Trimix_Enclosure_A1 (Autodesk Fusion 360 design; units mm, degrees)
Autodesk Fusion 360 part; units mm, degrees
(part 1 of 3)
ref_plane "WorkPlane1" through (0, 0, 0) normal (0, 0, 1) x (1, 0, 0) in component "01 Main housing"
sketch "Main housing sketch" plane through (0, 0, 0) normal (0, 0, 1) x (1, 0, 0) in component "01 Main housing"
  line L0 (-47.5, 0) -> (47.5, 0)
  line L1 (47.5, 0) -> (47.5, 180)
  line L2 (47.5, 180) -> (-47.5, 180)
  line L3 (-47.5, 180) -> (-47.5, 0)
  dimension "d42" = 47.5
  dimension "d43" = 95
  dimension "d44" = 180
  constraint horizontal origin L0.start
  constraint horizontal L0
  constraint vertical L1
  constraint horizontal L2
  constraint vertical L3
  measures "d42" horizontal distance of origin L0.start
  measures "d43" horizontal distance of L0.start L0.end
  measures "d44" vertical distance of L0.end L1.end
extrude "Main housing" add sketch "Main housing sketch" along normal blind 57 makes body 1 in component "01 Main housing"
fillet "Outside corner rounds" radius 8 4 edges at (-47.5, 180, 28.5) (47.5, 180, 28.5) (47.5, 0, 28.5) (-47.5, 0, 28.5) on bodies 1 in component "01 Main housing"
ref_plane "WorkPlane2" through (0, 0, 3) normal (0, 0, 1) x (1, 0, 0) in component "01 Main housing"
sketch "Rear-open cavity sketch" plane through (0, 0, 3) normal (0, 0, 1) x (1, 0, 0) in component "01 Main housing"
  line L0 (-44.5, 3) -> (44.5, 3)
  line L1 (44.5, 3) -> (44.5, 177)
  line L2 (44.5, 177) -> (-44.5, 177)
  line L3 (-44.5, 177) -> (-44.5, 3)
  dimension "d51" = 44.5
  dimension "d52" = 3
  dimension "d53" = 89
  dimension "d54" = 174
  constraint horizontal L0
  constraint vertical L1
  constraint horizontal L2
  constraint vertical L3
  measures "d51" horizontal distance of origin L0.start
  measures "d52" vertical distance of origin L0.start
  measures "d53" horizontal distance of L0.start L0.end
  measures "d54" vertical distance of L0.end L1.end
extrude "Rear-open cavity" cut sketch "Rear-open cavity sketch" along normal blind 60 bodies 1 in component "01 Main housing"
fillet "Inside corner rounds" radius 5 4 edges at (44.5, 3, 30) (-44.5, 3, 30) (-44.5, 177, 30) (44.5, 177, 30) on bodies 1 in component "01 Main housing"
ref_plane "WorkPlane3" through (0, 0, -1) normal (0, 0, 1) x (1, 0, 0) in component "01 Main housing"
sketch "Screen aperture sketch" plane through (0, 0, -1) normal (0, 0, 1) x (1, 0, 0) in component "01 Main housing"
  line L0 (-28.58, 21.205) -> (28.58, 21.205)
  line L1 (28.58, 21.205) -> (28.58, 115.805)
  line L2 (28.58, 115.805) -> (-28.58, 115.805)
  line L3 (-28.58, 115.805) -> (-28.58, 21.205)
  dimension "d61" = 28.58
  dimension "d62" = 21.205
  dimension "d63" = 57.16
  dimension "d64" = 94.6
  constraint horizontal L0
  constraint vertical L1
  constraint horizontal L2
  constraint vertical L3
  measures "d61" horizontal distance of origin L0.start
  measures "d62" vertical distance of origin L0.start
  measures "d63" horizontal distance of L0.start L0.end
  measures "d64" vertical distance of L0.end L1.end
extrude "Screen aperture" cut sketch "Screen aperture sketch" along normal blind 5 bodies 1 in component "01 Main housing"
ref_plane "WorkPlane4" through (0, 0, 3) normal (0, 0, 1) x (1, 0, 0) in component "01 Main housing"
sketch "Boss -1_0 sketch" plane through (0, 0, 3) normal (0, 0, 1) x (1, 0, 0) in component "01 Main housing"
  circle A0 centre (-40, 8) radius 4.5
  dimension "d69" = 40
  dimension "d70" = 8
  dimension "d71" = 4.5
  measures "d69" horizontal distance of origin A0.centre
  measures "d70" vertical distance of origin A0.centre
  measures "d71" radius of A0
extrude "Boss -1_0" add sketch "Boss -1_0 sketch" along normal blind 54 bodies 1 in component "01 Main housing"
ref_plane "WorkPlane5" through (0, 0, 3) normal (0, 0, 1) x (1, 0, 0) in component "01 Main housing"
sketch "Boss web -1_0 sketch" plane through (0, 0, 3) normal (0, 0, 1) x (1, 0, 0) in component "01 Main housing"
  line L0 (-44.5, 3.5) -> (-40, 3.5)
  line L1 (-40, 3.5) -> (-40, 12.5)
  line L2 (-40, 12.5) -> (-44.5, 12.5)
  line L3 (-44.5, 12.5) -> (-44.5, 3.5)
  dimension "d76" = 44.5
  dimension "d77" = 3.5
  dimension "d78" = 4.5
  dimension "d79" = 9
  constraint horizontal L0
  constraint vertical L1
  constraint horizontal L2
  constraint vertical L3
  measures "d76" horizontal distance of origin L0.start
  measures "d77" vertical distance of origin L0.start
  measures "d78" horizontal distance of L0.start L0.end
  measures "d79" vertical distance of L0.end L1.end
extrude "Boss web -1_0" add sketch "Boss web -1_0 sketch" along normal blind 54 bodies 1 in component "01 Main housing"
ref_plane "WorkPlane6" through (0, 0, 52) normal (0, 0, 1) x (1, 0, 0) in component "01 Main housing"
sketch "Insert pilot -1_0 sketch" plane through (0, 0, 52) normal (0, 0, 1) x (1, 0, 0) in component "01 Main housing"
  circle A0 centre (-40, 8) radius 2.1
  dimension "d84" = 40
  dimension "d85" = 8
  dimension "d86" = 2.1
  measures "d84" horizontal distance of origin A0.centre
  measures "d85" vertical distance of origin A0.centre
  measures "d86" radius of A0
extrude "Insert pilot -1_0" cut sketch "Insert pilot -1_0 sketch" along normal blind 5.1 bodies 1 in component "01 Main housing"
ref_plane "WorkPlane7" through (0, 0, 3) normal (0, 0, 1) x (1, 0, 0) in component "01 Main housing"
sketch "Boss -1_1 sketch" plane through (0, 0, 3) normal (0, 0, 1) x (1, 0, 0) in component "01 Main housing"
  circle A0 centre (-40, 90) radius 4.5
  dimension "d91" = 40
  dimension "d92" = 90
  dimension "d93" = 4.5
  measures "d91" horizontal distance of origin A0.centre
  measures "d92" vertical distance of origin A0.centre
  measures "d93" radius of A0
extrude "Boss -1_1" add sketch "Boss -1_1 sketch" along normal blind 54 bodies 1 in component "01 Main housing"
ref_plane "WorkPlane8" through (0, 0, 3) normal (0, 0, 1) x (1, 0, 0) in component "01 Main housing"
sketch "Boss web -1_1 sketch" plane through (0, 0, 3) normal (0, 0, 1) x (1, 0, 0) in component "01 Main housing"
  line L0 (-44.5, 85.5) -> (-40, 85.5)
  line L1 (-40, 85.5) -> (-40, 94.5)
  line L2 (-40, 94.5) -> (-44.5, 94.5)
  line L3 (-44.5, 94.5) -> (-44.5, 85.5)
  dimension "d98" = 44.5
  dimension "d99" = 85.5
  dimension "d100" = 4.5
  dimension "d101" = 9
  constraint horizontal L0
  constraint vertical L1
  constraint horizontal L2
  constraint vertical L3
  measures "d98" horizontal distance of origin L0.start
  measures "d99" vertical distance of origin L0.start
  measures "d100" horizontal distance of L0.start L0.end
  measures "d101" vertical distance of L0.end L1.end
extrude "Boss web -1_1" add sketch "Boss web -1_1 sketch" along normal blind 54 bodies 1 in component "01 Main housing"
ref_plane "WorkPlane9" through (0, 0, 52) normal (0, 0, 1) x (1, 0, 0) in component "01 Main housing"
sketch "Insert pilot -1_1 sketch" plane through (0, 0, 52) normal (0, 0, 1) x (1, 0, 0) in component "01 Main housing"
  circle A0 centre (-40, 90) radius 2.1
  dimension "d106" = 40
  dimension "d107" = 90
  dimension "d108" = 2.1
  measures "d106" horizontal distance of origin A0.centre
  measures "d107" vertical distance of origin A0.centre
  measures "d108" radius of A0
extrude "Insert pilot -1_1" cut sketch "Insert pilot -1_1 sketch" along normal blind 5.1 bodies 1 in component "01 Main housing"
ref_plane "WorkPlane10" through (0, 0, 3) normal (0, 0, 1) x (1, 0, 0) in component "01 Main housing"
sketch "Boss -1_2 sketch" plane through (0, 0, 3) normal (0, 0, 1) x (1, 0, 0) in component "01 Main housing"
  circle A0 centre (-40, 172) radius 4.5
  dimension "d113" = 40
  dimension "d114" = 172
  dimension "d115" = 4.5
  measures "d113" horizontal distance of origin A0.centre
  measures "d114" vertical distance of origin A0.centre
  measures "d115" radius of A0
extrude "Boss -1_2" add sketch "Boss -1_2 sketch" along normal blind 54 bodies 1 in component "01 Main housing"
ref_plane "WorkPlane11" through (0, 0, 3) normal (0, 0, 1) x (1, 0, 0) in component "01 Main housing"
sketch "Boss web -1_2 sketch" plane through (0, 0, 3) normal (0, 0, 1) x (1, 0, 0) in component "01 Main housing"
  line L0 (-44.5, 167.5) -> (-40, 167.5)
  line L1 (-40, 167.5) -> (-40, 176.5)
  line L2 (-40, 176.5) -> (-44.5, 176.5)
  line L3 (-44.5, 176.5) -> (-44.5, 167.5)
  dimension "d120" = 44.5
  dimension "d121" = 167.5
  dimension "d122" = 4.5
  dimension "d123" = 9
  constraint horizontal L0
  constraint vertical L1
  constraint horizontal L2
  constraint vertical L3
  measures "d120" horizontal distance of origin L0.start
  measures "d121" vertical distance of origin L0.start
  measures "d122" horizontal distance of L0.start L0.end
  measures "d123" vertical distance of L0.end L1.end
extrude "Boss web -1_2" add sketch "Boss web -1_2 sketch" along normal blind 54 bodies 1 in component "01 Main housing"
ref_plane "WorkPlane12" through (0, 0, 52) normal (0, 0, 1) x (1, 0, 0) in component "01 Main housing"
sketch "Insert pilot -1_2 sketch" plane through (0, 0, 52) normal (0, 0, 1) x (1, 0, 0) in component "01 Main housing"
  circle A0 centre (-40, 172) radius 2.1
  dimension "d128" = 40
  dimension "d129" = 172
  dimension "d130" = 2.1
  measures "d128" horizontal distance of origin A0.centre
  measures "d129" vertical distance of origin A0.centre
  measures "d130" radius of A0
extrude "Insert pilot -1_2" cut sketch "Insert pilot -1_2 sketch" along normal blind 5.1 bodies 1 in component "01 Main housing"
ref_plane "WorkPlane13" through (0, 0, 3) normal (0, 0, 1) x (1, 0, 0) in component "01 Main housing"
sketch "Boss 1_0 sketch" plane through (0, 0, 3) normal (0, 0, 1) x (1, 0, 0) in component "01 Main housing"
  circle A0 centre (40, 8) radius 4.5
  dimension "d135" = 40
  dimension "d136" = 8
  dimension "d137" = 4.5
  measures "d135" horizontal distance of origin A0.centre
  measures "d136" vertical distance of origin A0.centre
  measures "d137" radius of A0
extrude "Boss 1_0" add sketch "Boss 1_0 sketch" along normal blind 54 bodies 1 in component "01 Main housing"
ref_plane "WorkPlane14" through (0, 0, 3) normal (0, 0, 1) x (1, 0, 0) in component "01 Main housing"
sketch "Boss web 1_0 sketch" plane through (0, 0, 3) normal (0, 0, 1) x (1, 0, 0) in component "01 Main housing"
  line L0 (40, 3.5) -> (44.5, 3.5)
  line L1 (44.5, 3.5) -> (44.5, 12.5)
  line L2 (44.5, 12.5) -> (40, 12.5)
  line L3 (40, 12.5) -> (40, 3.5)
  dimension "d142" = 40
  dimension "d143" = 3.5
  dimension "d144" = 4.5
  dimension "d145" = 9
  constraint horizontal L0
  constraint vertical L1
  constraint horizontal L2
  constraint vertical L3
  measures "d142" horizontal distance of origin L0.start
  measures "d143" vertical distance of origin L0.start
  measures "d144" horizontal distance of L0.start L0.end
  measures "d145" vertical distance of L0.end L1.end
extrude "Boss web 1_0" add sketch "Boss web 1_0 sketch" along normal blind 54 bodies 1 in component "01 Main housing"
ref_plane "WorkPlane15" through (0, 0, 52) normal (0, 0, 1) x (1, 0, 0) in component "01 Main housing"
sketch "Insert pilot 1_0 sketch" plane through (0, 0, 52) normal (0, 0, 1) x (1, 0, 0) in component "01 Main housing"
  circle A0 centre (40, 8) radius 2.1
  dimension "d150" = 40
  dimension "d151" = 8
  dimension "d152" = 2.1
  measures "d150" horizontal distance of origin A0.centre
  measures "d151" vertical distance of origin A0.centre
  measures "d152" radius of A0
extrude "Insert pilot 1_0" cut sketch "Insert pilot 1_0 sketch" along normal blind 5.1 bodies 1 in component "01 Main housing"
ref_plane "WorkPlane16" through (0, 0, 3) normal (0, 0, 1) x (1, 0, 0) in component "01 Main housing"
sketch "Boss 1_1 sketch" plane through (0, 0, 3) normal (0, 0, 1) x (1, 0, 0) in component "01 Main housing"
  circle A0 centre (40, 90) radius 4.5
  dimension "d157" = 40
  dimension "d158" = 90
  dimension "d159" = 4.5
  measures "d157" horizontal distance of origin A0.centre
  measures "d158" vertical distance of origin A0.centre
  measures "d159" radius of A0
extrude "Boss 1_1" add sketch "Boss 1_1 sketch" along normal blind 54 bodies 1 in component "01 Main housing"
ref_plane "WorkPlane17" through (0, 0, 3) normal (0, 0, 1) x (1, 0, 0) in component "01 Main housing"
sketch "Boss web 1_1 sketch" plane through (0, 0, 3) normal (0, 0, 1) x (1, 0, 0) in component "01 Main housing"
  line L0 (40, 85.5) -> (44.5, 85.5)
  line L1 (44.5, 85.5) -> (44.5, 94.5)
  line L2 (44.5, 94.5) -> (40, 94.5)
  line L3 (40, 94.5) -> (40, 85.5)
  dimension "d164" = 40
  dimension "d165" = 85.5
  dimension "d166" = 4.5
  dimension "d167" = 9
  constraint horizontal L0
  constraint vertical L1
  constraint horizontal L2
  constraint vertical L3
  measures "d164" horizontal distance of origin L0.start
  measures "d165" vertical distance of origin L0.start
  measures "d166" horizontal distance of L0.start L0.end
  measures "d167" vertical distance of L0.end L1.end
extrude "Boss web 1_1" add sketch "Boss web 1_1 sketch" along normal blind 54 bodies 1 in component "01 Main housing"
ref_plane "WorkPlane18" through (0, 0, 52) normal (0, 0, 1) x (1, 0, 0) in component "01 Main housing"
sketch "Insert pilot 1_1 sketch" plane through (0, 0, 52) normal (0, 0, 1) x (1, 0, 0) in component "01 Main housing"
  circle A0 centre (40, 90) radius 2.1
  dimension "d172" = 40
  dimension "d173" = 90
  dimension "d174" = 2.1
  measures "d172" horizontal distance of origin A0.centre
  measures "d173" vertical distance of origin A0.centre
  measures "d174" radius of A0
extrude "Insert pilot 1_1" cut sketch "Insert pilot 1_1 sketch" along normal blind 5.1 bodies 1 in component "01 Main housing"
ref_plane "WorkPlane19" through (0, 0, 3) normal (0, 0, 1) x (1, 0, 0) in component "01 Main housing"
sketch "Boss 1_2 sketch" plane through (0, 0, 3) normal (0, 0, 1) x (1, 0, 0) in component "01 Main housing"
  circle A0 centre (40, 172) radius 4.5
  dimension "d179" = 40
  dimension "d180" = 172
  dimension "d181" = 4.5
  measures "d179" horizontal distance of origin A0.centre
  measures "d180" vertical distance of origin A0.centre
  measures "d181" radius of A0
extrude "Boss 1_2" add sketch "Boss 1_2 sketch" along normal blind 54 bodies 1 in component "01 Main housing"
ref_plane "WorkPlane20" through (0, 0, 3) normal (0, 0, 1) x (1, 0, 0) in component "01 Main housing"
sketch "Boss web 1_2 sketch" plane through (0, 0, 3) normal (0, 0, 1) x (1, 0, 0) in component "01 Main housing"
  line L0 (40, 167.5) -> (44.5, 167.5)
  line L1 (44.5, 167.5) -> (44.5, 176.5)
  line L2 (44.5, 176.5) -> (40, 176.5)
  line L3 (40, 176.5) -> (40, 167.5)
  dimension "d186" = 40
  dimension "d187" = 167.5
  dimension "d188" = 4.5
  dimension "d189" = 9
  constraint horizontal L0
  constraint vertical L1
  constraint horizontal L2
  constraint vertical L3
  measures "d186" horizontal distance of origin L0.start
  measures "d187" vertical distance of origin L0.start
  measures "d188" horizontal distance of L0.start L0.end
  measures "d189" vertical distance of L0.end L1.end
extrude "Boss web 1_2" add sketch "Boss web 1_2 sketch" along normal blind 54 bodies 1 in component "01 Main housing"
ref_plane "WorkPlane21" through (0, 0, 52) normal (0, 0, 1) x (1, 0, 0) in component "01 Main housing"
sketch "Insert pilot 1_2 sketch" plane through (0, 0, 52) normal (0, 0, 1) x (1, 0, 0) in component "01 Main housing"
  circle A0 centre (40, 172) radius 2.1
  dimension "d194" = 40
  dimension "d195" = 172
  dimension "d196" = 2.1
  measures "d194" horizontal distance of origin A0.centre
  measures "d195" vertical distance of origin A0.centre
  measures "d196" radius of A0
extrude "Insert pilot 1_2" cut sketch "Insert pilot 1_2 sketch" along normal blind 5.1 bodies 1 in component "01 Main housing"
ref_plane "WorkPlane22" through (-48.5, 0, 0) normal (1, 0, 0) x (0, 1, 0) in component "01 Main housing"
sketch "Upper side gas passages sketch" plane through (-48.5, 0, 0) normal (1, 0, 0) x (0, 0, -1) in component "01 Main housing"
  circle A0 centre (-12, 153.5) radius 4.5
  dimension "d202" = 153.5
  dimension "d203" = 4.5
  measures "d202" vertical distance of origin A0.centre
  measures "d203" radius of A0
extrude "Upper side gas passages" cut sketch "Upper side gas passages sketch" along normal blind 97 bodies 1 in component "01 Main housing"
ref_plane "WorkPlane23" through (-48.5, 0, 0) normal (1, 0, 0) x (0, 1, 0) in component "01 Main housing"
sketch "Right power button mounting hole sketch" plane through (-48.5, 0, 0) normal (1, 0, 0) x (0, 0, -1) in component "01 Main housing"
  circle A0 centre (-42, 102) radius 6
  dimension "d209" = 102
  dimension "d210" = 6
  measures "d209" vertical distance of origin A0.centre
  measures "d210" radius of A0
extrude "Right power button mounting hole" cut sketch "Right power button mounting hole sketch" along normal blind 5 bodies 1 in component "01 Main housing"
ref_plane "WorkPlane24" through (43.5, 0, 0) normal (1, 0, 0) x (0, 1, 0) in component "01 Main housing"
sketch "Left USB service-insert opening sketch" plane through (43.5, 0, 0) normal (1, 0, 0) x (0, 0, -1) in component "01 Main housing"
  line L0 (-42, 58) -> (-26, 58)
  line L1 (-26, 58) -> (-26, 78)
  line L2 (-26, 78) -> (-42, 78)
  line L3 (-42, 78) -> (-42, 58)
  dimension "d215" = 42
  dimension "d216" = 58
  dimension "d217" = 16
  dimension "d218" = 20
  constraint horizontal L0
  constraint vertical L1
  constraint horizontal L2
  constraint vertical L3
  measures "d215" horizontal distance of origin L0.start
  measures "d216" vertical distance of origin L0.start
  measures "d217" horizontal distance of L0.start L0.end
  measures "d218" vertical distance of L0.end L1.end
extrude "Left USB service-insert opening" cut sketch "Left USB service-insert opening sketch" along normal blind 5 bodies 1 in component "01 Main housing"
ref_plane "WorkPlane1" through (0, 0, 57.25) normal (0, 0, 1) x (1, 0, 0) in component "02 Single rear cover"
sketch "Single rear cover sketch" plane through (0, 0, 57.25) normal (0, 0, 1) x (1, 0, 0) in component "02 Single rear cover"
  line L0 (-47.5, 0) -> (47.5, 0)
  line L1 (47.5, 0) -> (47.5, 180)
  line L2 (47.5, 180) -> (-47.5, 180)
  line L3 (-47.5, 180) -> (-47.5, 0)
  dimension "d223" = 47.5
  dimension "d224" = 95
  dimension "d225" = 180
  constraint horizontal origin L0.start
  constraint horizontal L0
  constraint vertical L1
  constraint horizontal L2
  constraint vertical L3
  measures "d223" horizontal distance of origin L0.start
  measures "d224" horizontal distance of L0.start L0.end
  measures "d225" vertical distance of L0.end L1.end
extrude "Single rear cover" add sketch "Single rear cover sketch" along normal blind 2.75 separate body makes body 2 in component "02 Single rear cover"
fillet "Cover corner rounds" radius 8 4 edges at (-47.5, 180, 58.625) (47.5, 180, 58.625) (47.5, 0, 58.625) (-47.5, 0, 58.625) on bodies 2 in component "02 Single rear cover"
ref_plane "WorkPlane2" through (0, 0, 57) normal (0, 0, 1) x (1, 0, 0) in component "02 Single rear cover"
sketch "M3 clearance -1_0 sketch" plane through (0, 0, 57) normal (0, 0, 1) x (1, 0, 0) in component "02 Single rear cover"
  circle A0 centre (-40, 8) radius 1.7
  dimension "d232" = 40
  dimension "d233" = 8
  dimension "d234" = 1.7
  measures "d232" horizontal distance of origin A0.centre
  measures "d233" vertical distance of origin A0.centre
  measures "d234" radius of A0
extrude "M3 clearance -1_0" cut sketch "M3 clearance -1_0 sketch" along normal blind 4 bodies 2 in component "02 Single rear cover"
ref_plane "WorkPlane3" through (0, 0, 57) normal (0, 0, 1) x (1, 0, 0) in component "02 Single rear cover"
sketch "M3 clearance -1_1 sketch" plane through (0, 0, 57) normal (0, 0, 1) x (1, 0, 0) in component "02 Single rear cover"
  circle A0 centre (-40, 90) radius 1.7
  dimension "d239" = 40
  dimension "d240" = 90
  dimension "d241" = 1.7
  measures "d239" horizontal distance of origin A0.centre
  measures "d240" vertical distance of origin A0.centre
  measures "d241" radius of A0
extrude "M3 clearance -1_1" cut sketch "M3 clearance -1_1 sketch" along normal blind 4 bodies 2 in component "02 Single rear cover"
ref_plane "WorkPlane4" through (0, 0, 57) normal (0, 0, 1) x (1, 0, 0) in component "02 Single rear cover"
sketch "M3 clearance -1_2 sketch" plane through (0, 0, 57) normal (0, 0, 1) x (1, 0, 0) in component "02 Single rear cover"
  circle A0 centre (-40, 172) radius 1.7
  dimension "d246" = 40
  dimension "d247" = 172
  dimension "d248" = 1.7
  measures "d246" horizontal distance of origin A0.centre
  measures "d247" vertical distance of origin A0.centre
  measures "d248" radius of A0
extrude "M3 clearance -1_2" cut sketch "M3 clearance -1_2 sketch" along normal blind 4 bodies 2 in component "02 Single rear cover"
ref_plane "WorkPlane5" through (0, 0, 57) normal (0, 0, 1) x (1, 0, 0) in component "02 Single rear cover"
sketch "M3 clearance 1_0 sketch" plane through (0, 0, 57) normal (0, 0, 1) x (1, 0, 0) in component "02 Single rear cover"
  circle A0 centre (40, 8) radius 1.7
  dimension "d253" = 40
  dimension "d254" = 8
  dimension "d255" = 1.7
  measures "d253" horizontal distance of origin A0.centre
  measures "d254" vertical distance of origin A0.centre
  measures "d255" radius of A0
extrude "M3 clearance 1_0" cut sketch "M3 clearance 1_0 sketch" along normal blind 4 bodies 2 in component "02 Single rear cover"
ref_plane "WorkPlane6" through (0, 0, 57) normal (0, 0, 1) x (1, 0, 0) in component "02 Single rear cover"
sketch "M3 clearance 1_1 sketch" plane through (0, 0, 57) normal (0, 0, 1) x (1, 0, 0) in component "02 Single rear cover"
  circle A0 centre (40, 90) radius 1.7
  dimension "d260" = 40
  dimension "d261" = 90
  dimension "d262" = 1.7
  measures "d260" horizontal distance of origin A0.centre
  measures "d261" vertical distance of origin A0.centre
  measures "d262" radius of A0
extrude "M3 clearance 1_1" cut sketch "M3 clearance 1_1 sketch" along normal blind 4 bodies 2 in component "02 Single rear cover"
ref_plane "WorkPlane7" through (0, 0, 57) normal (0, 0, 1) x (1, 0, 0) in component "02 Single rear cover"
sketch "M3 clearance 1_2 sketch" plane through (0, 0, 57) normal (0, 0, 1) x (1, 0, 0) in component "02 Single rear cover"
  circle A0 centre (40, 172) radius 1.7
  dimension "d267" = 40
  dimension "d268" = 172
  dimension "d269" = 1.7
  measures "d267" horizontal distance of origin A0.centre
  measures "d268" vertical distance of origin A0.centre
  measures "d269" radius of A0
extrude "M3 clearance 1_2" cut sketch "M3 clearance 1_2 sketch" along normal blind 4 bodies 2 in component "02 Single rear cover"
ref_plane "WorkPlane1" through (0, 0, 3.5) normal (0, 0, 1) x (1, 0, 0) in component "03 Removable sampling chamber"
sketch "Sampling chamber body sketch" plane through (0, 0, 3.5) normal (0, 0, 1) x (1, 0, 0) in component "03 Removable sampling chamber"
  line L0 (-35, 132) -> (35, 132)
  line L1 (35, 132) -> (35, 175)
  line L2 (35, 175) -> (-35, 175)
  line L3 (-35, 175) -> (-35, 132)
  dimension "d274" = 35
  dimension "d275" = 132
  dimension "d276" = 70
  dimension "d277" = 43
  constraint horizontal L0
  constraint vertical L1
  constraint horizontal L2
  constraint vertical L3
  measures "d274" horizontal distance of origin L0.start
  measures "d275" vertical distance of origin L0.start
  measures "d276" horizontal distance of L0.start L0.end
  measures "d277" vertical distance of L0.end L1.end
extrude "Sampling chamber body" add sketch "Sampling chamber body sketch" along normal blind 51 separate body makes body 3 in component "03 Removable sampling chamber"
ref_plane "WorkPlane2" through (0, 0, 5.5) normal (0, 0, 1) x (1, 0, 0) in component "03 Removable sampling chamber"
sketch "Chamber cavity sketch" plane through (0, 0, 5.5) normal (0, 0, 1) x (1, 0, 0) in component "03 Removable sampling chamber"
  line L0 (-33, 134) -> (33, 134)
  line L1 (33, 134) -> (33, 173)
  line L2 (33, 173) -> (-33, 173)
  line L3 (-33, 173) -> (-33, 134)
  dimension "d282" = 33
  dimension "d283" = 134
  dimension "d284" = 66
  dimension "d285" = 39
  constraint horizontal L0
  constraint vertical L1
  constraint horizontal L2
  constraint vertical L3
  measures "d282" horizontal distance of origin L0.start
  measures "d283" vertical distance of origin L0.start
  measures "d284" horizontal distance of L0.start L0.end
  measures "d285" vertical distance of L0.end L1.end
extrude "Chamber cavity" cut sketch "Chamber cavity sketch" along normal blind 53 bodies 3 in component "03 Removable sampling chamber"
ref_plane "WorkPlane3" through (-36, 0, 0) normal (1, 0, 0) x (0, 1, 0) in component "03 Removable sampling chamber"
sketch "Sketch3" plane through (-36, 0, 0) normal (1, 0, 0) x (0, 0, -1) in component "03 Removable sampling chamber"
  circle A0 centre (-12, 153.5) radius 4.1
  dimension "d291" = 153.5
  dimension "d292" = 4.1
  measures "d291" vertical distance of origin A0.centre
  measures "d292" radius of A0
extrude "Gas fitting clearance — seal TBD" cut sketch "Sketch3" along normal blind 72 bodies 3 in component "03 Removable sampling chamber"
ref_plane "WorkPlane4" through (0, 0, 5.5) normal (0, 0, 1) x (1, 0, 0) in component "03 Removable sampling chamber"
sketch "Internal lid boss sketch" plane through (0, 0, 5.5) normal (0, 0, 1) x (1, 0, 0) in component "03 Removable sampling chamber"
  circle A0 centre (-30, 136) radius 3
  dimension "d297" = 30
  dimension "d298" = 136
  dimension "d299" = 3
  measures "d297" horizontal distance of origin A0.centre
  measures "d298" vertical distance of origin A0.centre
  measures "d299" radius of A0
extrude "Internal lid boss" add sketch "Internal lid boss sketch" along normal blind 49 bodies 3 in component "03 Removable sampling chamber"
ref_plane "WorkPlane5" through (0, 0, 50.5) normal (0, 0, 1) x (1, 0, 0) in component "03 Removable sampling chamber"
sketch "Sketch5" plane through (0, 0, 50.5) normal (0, 0, 1) x (1, 0, 0) in component "03 Removable sampling chamber"
  circle A0 centre (-30, 136) radius 1.3
  dimension "d304" = 30
  dimension "d305" = 136
  dimension "d306" = 1.3
  measures "d304" horizontal distance of origin A0.centre
  measures "d305" vertical distance of origin A0.centre
  measures "d306" radius of A0
extrude "Internal lid pilot — M2 insert TBD" cut sketch "Sketch5" along normal blind 4.1 bodies 3 in component "03 Removable sampling chamber"
ref_plane "WorkPlane6" through (0, 0, 5.5) normal (0, 0, 1) x (1, 0, 0) in component "03 Removable sampling chamber"
sketch "Internal lid boss sketch (1)" plane through (0, 0, 5.5) normal (0, 0, 1) x (1, 0, 0) in component "03 Removable sampling chamber"
  circle A0 centre (-30, 171) radius 3
  dimension "d311" = 30
  dimension "d312" = 171
  dimension "d313" = 3
  measures "d311" horizontal distance of origin A0.centre
  measures "d312" vertical distance of origin A0.centre
  measures "d313" radius of A0
extrude "Internal lid boss (1)" add sketch "Internal lid boss sketch (1)" along normal blind 49 bodies 3 in component "03 Removable sampling chamber"
ref_plane "WorkPlane7" through (0, 0, 50.5) normal (0, 0, 1) x (1, 0, 0) in component "03 Removable sampling chamber"
sketch "Sketch7" plane through (0, 0, 50.5) normal (0, 0, 1) x (1, 0, 0) in component "03 Removable sampling chamber"
  circle A0 centre (-30, 171) radius 1.3
  dimension "d318" = 30
  dimension "d319" = 171
  dimension "d320" = 1.3
  measures "d318" horizontal distance of origin A0.centre
  measures "d319" vertical distance of origin A0.centre
  measures "d320" radius of A0
extrude "Internal lid pilot — M2 insert TBD (1)" cut sketch "Sketch7" along normal blind 4.1 bodies 3 in component "03 Removable sampling chamber"
ref_plane "WorkPlane8" through (0, 0, 5.5) normal (0, 0, 1) x (1, 0, 0) in component "03 Removable sampling chamber"
sketch "Internal lid boss sketch (2)" plane through (0, 0, 5.5) normal (0, 0, 1) x (1, 0, 0) in component "03 Removable sampling chamber"
  circle A0 centre (30, 136) radius 3
  dimension "d325" = 30
  dimension "d326" = 136
  dimension "d327" = 3
  measures "d325" horizontal distance of origin A0.centre
  measures "d326" vertical distance of origin A0.centre
  measures "d327" radius of A0
extrude "Internal lid boss (2)" add sketch "Internal lid boss sketch (2)" along normal blind 49 bodies 3 in component "03 Removable sampling chamber"
ref_plane "WorkPlane9" through (0, 0, 50.5) normal (0, 0, 1) x (1, 0, 0) in component "03 Removable sampling chamber"
sketch "Sketch9" plane through (0, 0, 50.5) normal (0, 0, 1) x (1, 0, 0) in component "03 Removable sampling chamber"
  circle A0 centre (30, 136) radius 1.3
  dimension "d332" = 30
  dimension "d333" = 136
  dimension "d334" = 1.3
  measures "d332" horizontal distance of origin A0.centre
  measures "d333" vertical distance of origin A0.centre
  measures "d334" radius of A0
extrude "Internal lid pilot — M2 insert TBD (2)" cut sketch "Sketch9" along normal blind 4.1 bodies 3 in component "03 Removable sampling chamber"
ref_plane "WorkPlane10" through (0, 0, 5.5) normal (0, 0, 1) x (1, 0, 0) in component "03 Removable sampling chamber"
sketch "Internal lid boss sketch (3)" plane through (0, 0, 5.5) normal (0, 0, 1) x (1, 0, 0) in component "03 Removable sampling chamber"
  circle A0 centre (30, 171) radius 3
  dimension "d339" = 30
  dimension "d340" = 171
  dimension "d341" = 3
  measures "d339" horizontal distance of origin A0.centre
  measures "d340" vertical distance of origin A0.centre
  measures "d341" radius of A0
extrude "Internal lid boss (3)" add sketch "Internal lid boss sketch (3)" along normal blind 49 bodies 3 in component "03 Removable sampling chamber"
ref_plane "WorkPlane11" through (0, 0, 50.5) normal (0, 0, 1) x (1, 0, 0) in component "03 Removable sampling chamber"
sketch "Sketch11" plane through (0, 0, 50.5) normal (0, 0, 1) x (1, 0, 0) in component "03 Removable sampling chamber"
  circle A0 centre (30, 171) radius 1.3
  dimension "d346" = 30
  dimension "d347" = 171
  dimension "d348" = 1.3
  measures "d346" horizontal distance of origin A0.centre
  measures "d347" vertical distance of origin A0.centre
  measures "d348" radius of A0
extrude "Internal lid pilot — M2 insert TBD (3)" cut sketch "Sketch11" along normal blind 4.1 bodies 3 in component "03 Removable sampling chamber"
ref_plane "WorkPlane12" through (0, 0, 47) normal (0, 0, 1) x (1, 0, 0) in component "03 Removable sampling chamber"
sketch "Cartridge attachment ear sketch" plane through (0, 0, 47) normal (0, 0, 1) x (1, 0, 0) in component "03 Removable sampling chamber"
  line L0 (-41, 134) -> (-34.5, 134)
  line L1 (-34.5, 134) -> (-34.5, 140)
  line L2 (-34.5, 140) -> (-41, 140)
  line L3 (-41, 140) -> (-41, 134)
  dimension "d353" = 41
  dimension "d354" = 134
  dimension "d355" = 6.5
  dimension "d356" = 6
  constraint horizontal L0
  constraint vertical L1
  constraint horizontal L2
  constraint vertical L3
  measures "d353" horizontal distance of origin L0.start
  measures "d354" vertical distance of origin L0.start
  measures "d355" horizontal distance of L0.start L0.end
  measures "d356" vertical distance of L0.end L1.end
extrude "Cartridge attachment ear" add sketch "Cartridge attachment ear sketch" along normal blind 3 bodies 3 in component "03 Removable sampling chamber"
ref_plane "WorkPlane13" through (0, 0, 46.9) normal (0, 0, 1) x (1, 0, 0) in component "03 Removable sampling chamber"
sketch "Cartridge clearance sketch" plane through (0, 0, 46.9) normal (0, 0, 1) x (1, 0, 0) in component "03 Removable sampling chamber"
  circle A0 centre (-38, 137) radius 1.2
  dimension "d361" = 38
  dimension "d362" = 137
  dimension "d363" = 1.2
  measures "d361" horizontal distance of origin A0.centre
  measures "d362" vertical distance of origin A0.centre
  measures "d363" radius of A0
extrude "Cartridge clearance" cut sketch "Cartridge clearance sketch" along normal blind 3.2 bodies 3 in component "03 Removable sampling chamber"
ref_plane "WorkPlane25" through (0, 0, 3) normal (0, 0, 1) x (1, 0, 0) in component "01 Main housing"
sketch "Cartridge support post sketch" plane through (0, 0, 3) normal (0, 0, 1) x (1, 0, 0) in component "01 Main housing"
  circle A0 centre (-38, 137) radius 2.5
  dimension "d368" = 38
  dimension "d369" = 137
  dimension "d370" = 2.5
  measures "d368" horizontal distance of origin A0.centre
  measures "d369" vertical distance of origin A0.centre
  measures "d370" radius of A0
extrude "Cartridge support post" add sketch "Cartridge support post sketch" along normal blind 44 bodies 1 in component "01 Main housing"
ref_plane "WorkPlane26" through (0, 0, 42) normal (0, 0, 1) x (1, 0, 0) in component "01 Main housing"
sketch "Sketch26" plane through (0, 0, 42) normal (0, 0, 1) x (1, 0, 0) in component "01 Main housing"
  circle A0 centre (-38, 137) radius 1.3
  dimension "d375" = 38
  dimension "d376" = 137
  dimension "d377" = 1.3
  measures "d375" horizontal distance of origin A0.centre
  measures "d376" vertical distance of origin A0.centre
  measures "d377" radius of A0
extrude "Cartridge support pilot — M3 TBD" cut sketch "Sketch26" along normal blind 5.1 bodies 1 in component "01 Main housing"
ref_plane "WorkPlane14" through (0, 0, 47) normal (0, 0, 1) x (1, 0, 0) in component "03 Removable sampling chamber"
sketch "Cartridge attachment ear sketch (1)" plane through (0, 0, 47) normal (0, 0, 1) x (1, 0, 0) in component "03 Removable sampling chamber"
  line L0 (-41, 160) -> (-34.5, 160)
  line L1 (-34.5, 160) -> (-34.5, 166)
  line L2 (-34.5, 166) -> (-41, 166)
  line L3 (-41, 166) -> (-41, 160)
  dimension "d382" = 41
  dimension "d383" = 160
  dimension "d384" = 6.5
  dimension "d385" = 6
  constraint horizontal L0
  constraint vertical L1
  constraint horizontal L2
  constraint vertical L3
  measures "d382" horizontal distance of origin L0.start
  measures "d383" vertical distance of origin L0.start
  measures "d384" horizontal distance of L0.start L0.end
  measures "d385" vertical distance of L0.end L1.end
extrude "Cartridge attachment ear (1)" add sketch "Cartridge attachment ear sketch (1)" along normal blind 3 bodies 3 in component "03 Removable sampling chamber"
ref_plane "WorkPlane15" through (0, 0, 46.9) normal (0, 0, 1) x (1, 0, 0) in component "03 Removable sampling chamber"
sketch "Cartridge clearance sketch (1)" plane through (0, 0, 46.9) normal (0, 0, 1) x (1, 0, 0) in component "03 Removable sampling chamber"
  circle A0 centre (-38, 163) radius 1.2
  dimension "d390" = 38
  dimension "d391" = 163
  dimension "d392" = 1.2
  measures "d390" horizontal distance of origin A0.centre
  measures "d391" vertical distance of origin A0.centre
  measures "d392" radius of A0
extrude "Cartridge clearance (1)" cut sketch "Cartridge clearance sketch (1)" along normal blind 3.2 bodies 3 in component "03 Removable sampling chamber"
ref_plane "WorkPlane27" through (0, 0, 3) normal (0, 0, 1) x (1, 0, 0) in component "01 Main housing"
sketch "Cartridge support post sketch (1)" plane through (0, 0, 3) normal (0, 0, 1) x (1, 0, 0) in component "01 Main housing"
  circle A0 centre (-38, 163) radius 2.5
  dimension "d397" = 38
  dimension "d398" = 163
  dimension "d399" = 2.5
  measures "d397" horizontal distance of origin A0.centre
  measures "d398" vertical distance of origin A0.centre
  measures "d399" radius of A0
extrude "Cartridge support post (1)" add sketch "Cartridge support post sketch (1)" along normal blind 44 bodies 1 in component "01 Main housing"
ref_plane "WorkPlane28" through (0, 0, 42) normal (0, 0, 1) x (1, 0, 0) in component "01 Main housing"
sketch "Sketch28" plane through (0, 0, 42) normal (0, 0, 1) x (1, 0, 0) in component "01 Main housing"
  circle A0 centre (-38, 163) radius 1.3
  dimension "d404" = 38
  dimension "d405" = 163
  dimension "d406" = 1.3
  measures "d404" horizontal distance of origin A0.centre
  measures "d405" vertical distance of origin A0.centre
  measures "d406" radius of A0
extrude "Cartridge support pilot — M3 TBD (1)" cut sketch "Sketch28" along normal blind 5.1 bodies 1 in component "01 Main housing"
ref_plane "WorkPlane16" through (0, 0, 47) normal (0, 0, 1) x (1, 0, 0) in component "03 Removable sampling chamber"
sketch "Cartridge attachment ear sketch (2)" plane through (0, 0, 47) normal (0, 0, 1) x (1, 0, 0) in component "03 Removable sampling chamber"
  line L0 (34.5, 134) -> (41, 134)
  line L1 (41, 134) -> (41, 140)
  line L2 (41, 140) -> (34.5, 140)
  line L3 (34.5, 140) -> (34.5, 134)
  dimension "d411" = 34.5
  dimension "d412" = 134
  dimension "d413" = 6.5
  dimension "d414" = 6
  constraint horizontal L0
  constraint vertical L1
  constraint horizontal L2
  constraint vertical L3
  measures "d411" horizontal distance of origin L0.start
  measures "d412" vertical distance of origin L0.start
  measures "d413" horizontal distance of L0.start L0.end
  measures "d414" vertical distance of L0.end L1.end
extrude "Cartridge attachment ear (2)" add sketch "Cartridge attachment ear sketch (2)" along normal blind 3 bodies 3 in component "03 Removable sampling chamber"
ref_plane "WorkPlane17" through (0, 0, 46.9) normal (0, 0, 1) x (1, 0, 0) in component "03 Removable sampling chamber"
sketch "Cartridge clearance sketch (2)" plane through (0, 0, 46.9) normal (0, 0, 1) x (1, 0, 0) in component "03 Removable sampling chamber"
  circle A0 centre (38, 137) radius 1.2
  dimension "d419" = 38
  dimension "d420" = 137
  dimension "d421" = 1.2
  measures "d419" horizontal distance of origin A0.centre
  measures "d420" vertical distance of origin A0.centre
  measures "d421" radius of A0
extrude "Cartridge clearance (2)" cut sketch "Cartridge clearance sketch (2)" along normal blind 3.2 bodies 3 in component "03 Removable sampling chamber"
ref_plane "WorkPlane29" through (0, 0, 3) normal (0, 0, 1) x (1, 0, 0) in component "01 Main housing"
sketch "Cartridge support post sketch (2)" plane through (0, 0, 3) normal (0, 0, 1) x (1, 0, 0) in component "01 Main housing"
  circle A0 centre (38, 137) radius 2.5
  dimension "d426" = 38
  dimension "d427" = 137
  dimension "d428" = 2.5
  measures "d426" horizontal distance of origin A0.centre
  measures "d427" vertical distance of origin A0.centre
  measures "d428" radius of A0
extrude "Cartridge support post (2)" add sketch "Cartridge support post sketch (2)" along normal blind 44 bodies 1 in component "01 Main housing"
ref_plane "WorkPlane30" through (0, 0, 42) normal (0, 0, 1) x (1, 0, 0) in component "01 Main housing"
sketch "Sketch30" plane through (0, 0, 42) normal (0, 0, 1) x (1, 0, 0) in component "01 Main housing"
  circle A0 centre (38, 137) radius 1.3
  dimension "d433" = 38
  dimension "d434" = 137
  dimension "d435" = 1.3
  measures "d433" horizontal distance of origin A0.centre
  measures "d434" vertical distance of origin A0.centre
  measures "d435" radius of A0
extrude "Cartridge support pilot — M3 TBD (2)" cut sketch "Sketch30" along normal blind 5.1 bodies 1 in component "01 Main housing"
ref_plane "WorkPlane18" through (0, 0, 47) normal (0, 0, 1) x (1, 0, 0) in component "03 Removable sampling chamber"
sketch "Cartridge attachment ear sketch (3)" plane through (0, 0, 47) normal (0, 0, 1) x (1, 0, 0) in component "03 Removable sampling chamber"
  line L0 (34.5, 160) -> (41, 160)
  line L1 (41, 160) -> (41, 166)
  line L2 (41, 166) -> (34.5, 166)
  line L3 (34.5, 166) -> (34.5, 160)
  dimension "d440" = 34.5
  dimension "d441" = 160
  dimension "d442" = 6.5
  dimension "d443" = 6
  constraint horizontal L0
  constraint vertical L1
  constraint horizontal L2
  constraint vertical L3
  measures "d440" horizontal distance of origin L0.start
  measures "d441" vertical distance of origin L0.start
  measures "d442" horizontal distance of L0.start L0.end
  measures "d443" vertical distance of L0.end L1.end
extrude "Cartridge attachment ear (3)" add sketch "Cartridge attachment ear sketch (3)" along normal blind 3 bodies 3 in component "03 Removable sampling chamber"
ref_plane "WorkPlane19" through (0, 0, 46.9) normal (0, 0, 1) x (1, 0, 0) in component "03 Removable sampling chamber"
sketch "Cartridge clearance sketch (3)" plane through (0, 0, 46.9) normal (0, 0, 1) x (1, 0, 0) in component "03 Removable sampling chamber"
  circle A0 centre (38, 163) radius 1.2
  dimension "d448" = 38
  dimension "d449" = 163
  dimension "d450" = 1.2
  measures "d448" horizontal distance of origin A0.centre
  measures "d449" vertical distance of origin A0.centre
  measures "d450" radius of A0
extrude "Cartridge clearance (3)" cut sketch "Cartridge clearance sketch (3)" along normal blind 3.2 bodies 3 in component "03 Removable sampling chamber"
ref_plane "WorkPlane31" through (0, 0, 3) normal (0, 0, 1) x (1, 0, 0) in component "01 Main housing"
sketch "Cartridge support post sketch (3)" plane through (0, 0, 3) normal (0, 0, 1) x (1, 0, 0) in component "01 Main housing"
  circle A0 centre (38, 163) radius 2.5
  dimension "d455" = 38
  dimension "d456" = 163
  dimension "d457" = 2.5
  measures "d455" horizontal distance of origin A0.centre
  measures "d456" vertical distance of origin A0.centre
  measures "d457" radius of A0
extrude "Cartridge support post (3)" add sketch "Cartridge support post sketch (3)" along normal blind 44 bodies 1 in component "01 Main housing"
ref_plane "WorkPlane32" through (0, 0, 42) normal (0, 0, 1) x (1, 0, 0) in component "01 Main housing"
sketch "Sketch32" plane through (0, 0, 42) normal (0, 0, 1) x (1, 0, 0) in component "01 Main housing"
  circle A0 centre (38, 163) radius 1.3
  dimension "d462" = 38
  dimension "d463" = 163
  dimension "d464" = 1.3
  measures "d462" horizontal distance of origin A0.centre
  measures "d463" vertical distance of origin A0.centre
  measures "d464" radius of A0
extrude "Cartridge support pilot — M3 TBD (3)" cut sketch "Sketch32" along normal blind 5.1 bodies 1 in component "01 Main housing"
ref_plane "WorkPlane1" through (0, 0, 54.5) normal (0, 0, 1) x (1, 0, 0) in component "04 Internal chamber lid"
sketch "Sketch1" plane through (0, 0, 54.5) normal (0, 0, 1) x (1, 0, 0) in component "04 Internal chamber lid"
  line L0 (-35, 132) -> (35, 132)
  line L1 (35, 132) -> (35, 175)
  line L2 (35, 175) -> (-35, 175)
  line L3 (-35, 175) -> (-35, 132)
  dimension "d469" = 35
  dimension "d470" = 132
  dimension "d471" = 70
  dimension "d472" = 43
  constraint horizontal L0
  constraint vertical L1
  constraint horizontal L2
  constraint vertical L3
  measures "d469" horizontal distance of origin L0.start
  measures "d470" vertical distance of origin L0.start
  measures "d471" horizontal distance of L0.start L0.end
  measures "d472" vertical distance of L0.end L1.end
extrude "Internal chamber lid — gasket groove TBD" add sketch "Sketch1" along normal blind 2 separate body makes body 4 in component "04 Internal chamber lid"
ref_plane "WorkPlane2" through (0, 0, 54.4) normal (0, 0, 1) x (1, 0, 0) in component "04 Internal chamber lid"
sketch "Internal lid M2 clearance sketch" plane through (0, 0, 54.4) normal (0, 0, 1) x (1, 0, 0) in component "04 Internal chamber lid"
  circle A0 centre (-30, 136) radius 1.2
  dimension "d477" = 30
  dimension "d478" = 136
  dimension "d479" = 1.2
  measures "d477" horizontal distance of origin A0.centre
  measures "d478" vertical distance of origin A0.centre
  measures "d479" radius of A0
extrude "Internal lid M2 clearance" cut sketch "Internal lid M2 clearance sketch" along normal blind 2.2 bodies 4 in component "04 Internal chamber lid"
ref_plane "WorkPlane3" through (0, 0, 54.4) normal (0, 0, 1) x (1, 0, 0) in component "04 Internal chamber lid"
sketch "Internal lid M2 clearance sketch (1)" plane through (0, 0, 54.4) normal (0, 0, 1) x (1, 0, 0) in component "04 Internal chamber lid"
  circle A0 centre (-30, 171) radius 1.2
  dimension "d484" = 30
  dimension "d485" = 171
  dimension "d486" = 1.2
  measures "d484" horizontal distance of origin A0.centre
  measures "d485" vertical distance of origin A0.centre
  measures "d486" radius of A0
extrude "Internal lid M2 clearance (1)" cut sketch "Internal lid M2 clearance sketch (1)" along normal blind 2.2 bodies 4 in component "04 Internal chamber lid"
ref_plane "WorkPlane4" through (0, 0, 54.4) normal (0, 0, 1) x (1, 0, 0) in component "04 Internal chamber lid"
sketch "Internal lid M2 clearance sketch (2)" plane through (0, 0, 54.4) normal (0, 0, 1) x (1, 0, 0) in component "04 Internal chamber lid"
  circle A0 centre (30, 136) radius 1.2
  dimension "d491" = 30
  dimension "d492" = 136
  dimension "d493" = 1.2
  measures "d491" horizontal distance of origin A0.centre
  measures "d492" vertical distance of origin A0.centre
  measures "d493" radius of A0
extrude "Internal lid M2 clearance (2)" cut sketch "Internal lid M2 clearance sketch (2)" along normal blind 2.2 bodies 4 in component "04 Internal chamber lid"
ref_plane "WorkPlane5" through (0, 0, 54.4) normal (0, 0, 1) x (1, 0, 0) in component "04 Internal chamber lid"
sketch "Internal lid M2 clearance sketch (3)" plane through (0, 0, 54.4) normal (0, 0, 1) x (1, 0, 0) in component "04 Internal chamber lid"
  circle A0 centre (30, 171) radius 1.2
  dimension "d498" = 30
  dimension "d499" = 171
  dimension "d500" = 1.2
  measures "d498" horizontal distance of origin A0.centre
  measures "d499" vertical distance of origin A0.centre
  measures "d500" radius of A0
extrude "Internal lid M2 clearance (3)" cut sketch "Internal lid M2 clearance sketch (3)" along normal blind 2.2 bodies 4 in component "04 Internal chamber lid"
ref_plane "WorkPlane20" through (0, 131.9, 0) normal (0, 1, 0) x (0, 0, 1) in component "03 Removable sampling chamber"
sketch "Sealed wire feedthrough opening" plane through (0, 131.9, 0) normal (0, 1, 0) x (1, 0, 0) in component "03 Removable sampling chamber"
  line L0 (-5, -53) -> (5, -53)
  line L1 (5, -53) -> (5, -48)
  line L2 (5, -48) -> (-5, -48)
  line L3 (-5, -48) -> (-5, -53)
  dimension "d505" = 5
  dimension "d506" = 53
  dimension "d507" = 10
  dimension "d508" = 5
  constraint horizontal L0
  constraint vertical L1
  constraint horizontal L2
  constraint vertical L3
  measures "d505" horizontal distance of origin L0.start
  measures "d506" vertical distance of origin L0.start
  measures "d507" horizontal distance of L0.start L0.end
  measures "d508" vertical distance of L0.end L1.end
extrude "Wire feedthrough cut" cut sketch "Sealed wire feedthrough opening" along normal blind 2.2 bodies 3 in component "03 Removable sampling chamber"
ref_plane "WorkPlane1" through (0, 0, 48) normal (0, 0, 1) x (1, 0, 0) in component "05 Feedthrough seal envelope TBD"
sketch "Potted wire seal envelope TBD sketch" plane through (0, 0, 48) normal (0, 0, 1) x (1, 0, 0) in component "05 Feedthrough seal envelope TBD"
  line L0 (-5, 132) -> (5, 132)
  line L1 (5, 132) -> (5, 134)
  line L2 (5, 134) -> (-5, 134)
  line L3 (-5, 134) -> (-5, 132)
  dimension "d513" = 5
  dimension "d514" = 132
  dimension "d515" = 10
  dimension "d516" = 2
  constraint horizontal L0
  constraint vertical L1
  constraint horizontal L2
  constraint vertical L3
  measures "d513" horizontal distance of origin L0.start
  measures "d514" vertical distance of origin L0.start
  measures "d515" horizontal distance of L0.start L0.end
  measures "d516" vertical distance of L0.end L1.end
extrude "Potted wire seal envelope TBD" add sketch "Potted wire seal envelope TBD sketch" along normal blind 5 separate body makes body 5 in component "05 Feedthrough seal envelope TBD"
ref_plane "WorkPlane1" through (-53.5, 0, 0) normal (1, 0, 0) x (0, 1, 0) in component "06 Gas fitting envelopes TBD"
sketch "Right exhaust fitting envelope sketch (1)" plane through (-53.5, 0, 0) normal (1, 0, 0) x (0, 0, -1) in component "06 Gas fitting envelopes TBD"
  circle A0 centre (-12, 153.5) radius 4
  dimension "d522" = 153.5
  dimension "d523" = 4
  measures "d522" vertical distance of origin A0.centre
  measures "d523" radius of A0
extrude "Right exhaust fitting envelope (1)" add sketch "Right exhaust fitting envelope sketch (1)" along normal blind 20.5 separate body makes body 6 in component "06 Gas fitting envelopes TBD"
ref_plane "WorkPlane2" through (-53.5, 0, 0) normal (1, 0, 0) x (0, 1, 0) in component "06 Gas fitting envelopes TBD"
sketch "Right exhaust bore sketch (1)" plane through (-53.5, 0, 0) normal (1, 0, 0) x (0, 0, -1) in component "06 Gas fitting envelopes TBD"
  circle A0 centre (-12, 153.5) radius 2.5
  dimension "d529" = 153.5
  dimension "d530" = 2.5
  measures "d529" vertical distance of origin A0.centre
  measures "d530" radius of A0
extrude "Right exhaust bore (1)" cut sketch "Right exhaust bore sketch (1)" along normal blind 20.5 bodies 6 in component "06 Gas fitting envelopes TBD"
ref_plane "WorkPlane3" through (33, 0, 0) normal (1, 0, 0) x (0, 1, 0) in component "06 Gas fitting envelopes TBD"
sketch "Left inlet fitting envelope sketch" plane through (33, 0, 0) normal (1, 0, 0) x (0, 0, -1) in component "06 Gas fitting envelopes TBD"
  circle A0 centre (-12, 153.5) radius 4
  dimension "d536" = 153.5
  dimension "d537" = 4
  measures "d536" vertical distance of origin A0.centre
  measures "d537" radius of A0
extrude "Left inlet fitting envelope" add sketch "Left inlet fitting envelope sketch" along normal blind 20.5 separate body makes body 7 in component "06 Gas fitting envelopes TBD"
ref_plane "WorkPlane4" through (33, 0, 0) normal (1, 0, 0) x (0, 1, 0) in component "06 Gas fitting envelopes TBD"
sketch "Left inlet bore sketch" plane through (33, 0, 0) normal (1, 0, 0) x (0, 0, -1) in component "06 Gas fitting envelopes TBD"
  circle A0 centre (-12, 153.5) radius 2.5
  dimension "d543" = 153.5
  dimension "d544" = 2.5
  measures "d543" vertical distance of origin A0.centre
  measures "d544" radius of A0